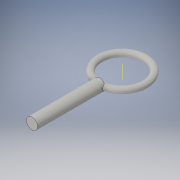
# Autodesk Inventor part: catapultLoop
Saved by Autodesk Inventor 2016 SP1 (Build 200210100, 210)
## iProperties
Created: 2016-01-16
Part Number: catapultLoop
Material: Generic
Document SubType Name: Modeling
Designer: steele
Density: 1 g/cm^3
Appearance: Default
Author: steele
Autodesk Inventor part; units mm, degrees
ref_plane "YZ Plane" through (0, 0, 0) normal (1, 0, 0) x (0, 1, 0)
ref_plane "XZ Plane" through (0, 0, 0) normal (0, 1, 0) x (-1, 0, 0)
sketch "Sketch3" plane through (0, 0, 0) normal (1, 0, 0) x (0, 1, 0)
  circle A0 centre (0, -101.6) radius 13.97
  line L0 (-19.558, 0) -> (19.558, 0) projected
  circle A1 centre (0, -101.6) radius 9.525
  point P0 (0, 0)
  dimension "d6" = 27.94
  dimension "d7" = 101.6
  dimension "d13" = 19.05
  constraints: 2 centre point, 1 coincident
  measures "d6" diameter of A0
  measures "d7" distance of point (0, 0) A0.centre
  measures "d13" diameter of A1
revolve "Revolution2" add sketch "Sketch3" angle 360 about axis through (0, -10, 0) along (0, 1, 0)
ref_plane "Work Plane2" through (0, 0, 101.6) normal (0, 0, 1) x (1, 0, 0)
sketch "Sketch4" plane through (0, 0, 101.6) normal (0, 0, 1) x (1, 0, 0)
  circle A0 centre (0, 0) radius 25.4
  dimension "d10" = 50.8
  constraints: 1 centre point, 1 coincident
  measures "d10" diameter of A0
extrude "Extrusion1" add sketch "Sketch4" along normal blind 304.8
equation "\"d6\" = ballHolderPipeOutsideDiam"
equation "\"d7\" = 0.5 * ballHolderLoopDiam"
equation "\"d13\" = ballHolderPipeInsideDiam"
equation "\"ballHolderLoopDiam\" = 203.2"
equation "\"ballHolderLoopHandleLength\" = 152.4"
equation "\"xxx\" = 0.5 * ballHolderLoopDiam + ballHolderLoopHandleLength"
equation "\"d9\" = 0.5 * ballHolderLoopDiam"
equation "\"ballHolderPipeInsideDiam\" = 19.05"
equation "\"ballHolderPipeOutsideDiam\" = 27.94"
equation "\"ballHolderLoopRadius\" = 0.5 * ballHolderLoopDiam"
body "Solid1"
